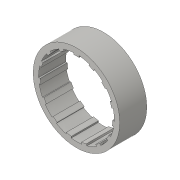
# Autodesk Inventor part: RubberWheelNT
Saved by Autodesk Inventor 2016 (Build 200138000, 138)
## iProperties
Created: 2016-01-25
Part Number: RubberWheelNT
Material: Generic
Document SubType Name: Modeling
Designer: 301278
Density: 1 g/cm^3
Appearance: Default
Author: 301278
Autodesk Inventor part; units mm, degrees
ref_plane "YZ Plane" through (0, 0, 0) normal (1, 0, 0) x (0, 1, 0)
ref_plane "XZ Plane" through (0, 0, 0) normal (0, 1, 0) x (-1, 0, 0)
ref_plane "XY Plane" through (0, 0, 0) normal (0, 0, 1) x (1, 0, 0)
sketch "Sketch1" plane through (0, 0, 0) normal (0, 0, 1) x (1, 0, 0)
  circle A0 centre (0, 0) radius 20.32
  circle A1 centre (0, 0) radius 17.78
  arc A2 (1.1871, 16.9765) -> (-1.1871, 16.9765) centre (0, 0) ccw
  line L0 (0, 17.018) -> (0, 20.32)
  line L1 (1.1871, 16.9765) -> (1.2403, 17.7367)
  line L2 (-1.1871, 16.9765) -> (-1.2403, 17.7367)
  dimension "d0" = 40.64
  dimension "d1" = 2.54
  dimension "d2" = 0.762
  dimension "d3" = 4
  dimension "d4" = 4
  constraints: 6 end point, 5 point on circle, 3 coincident, 2 centre point, 1 vertical, 1 vertical alignment, 2 other
  measures "d2" radial gap between concentric circles of A2 A1
  measures "d3" angle of L0 L2
  measures "d4" angle of L0 L1
extrude "Extrusion1" add sketch "Sketch1" along normal blind 12.7 contours A1 L1 A2 L0 | L0 A2 L2 A1 | A0
pattern_circular "Circular Pattern1" count 15 over 360 about axis through (0, 0, 0) along (0, 0, 1) of "Extrusion1"
body "Solid1"
